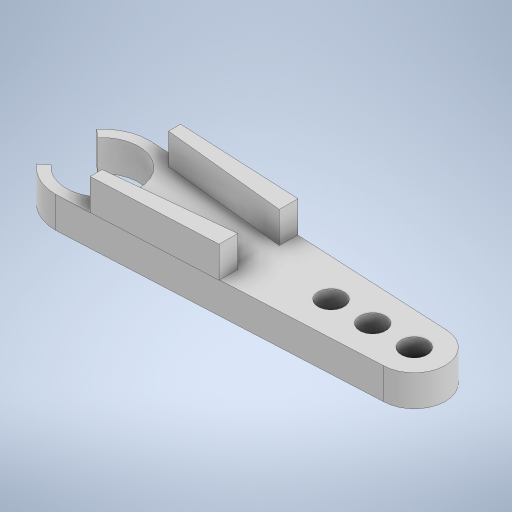
# Autodesk Inventor part: Servo Extension Clip-on
Saved by Autodesk Inventor 2023 (Build 270158000, 158)
## iProperties
Created: 2023-05-02
Part Number: Servo Extension Clip-on
Material: Generic
Document SubType Name: Modeling
Designer: adity
Density: 1 g/cm^3
Appearance: Default
Author: adity
Autodesk Inventor part; units mm, degrees
ref_plane "YZ Plane" through (0, 0, 0) normal (1, 0, 0) x (0, 1, 0)
ref_plane "XZ Plane" through (0, 0, 0) normal (0, 1, 0) x (-1, 0, 0)
ref_plane "XY Plane" through (0, 0, 0) normal (0, 0, 1) x (1, 0, 0)
sketch "Sketch2" plane through (0, 0, 0) normal (0, 1, 0) x (-1, 0, 0)
  circle A0 centre (0, 0) radius 3.5
  circle A1 centre (0, 0) radius 4.5
  line L0 (0, 0) -> (3.4472, 2.8925)
  line L1 (0, 0) -> (4.5, 0) construction
  line L2 (0, 0) -> (3.4472, -2.8925)
  line L3 (0, 0) -> (4.5, 0) construction
  line L4 (0, 0) -> (-30, 0)
  line L5 (0, 0) -> (30, 0) construction
  circle A2 centre (-30, 0) radius 1.25
  circle A3 centre (-26, 0) radius 1.25
  circle A4 centre (-22, 0) radius 1.25
  circle A5 centre (-30, 0) radius 3
  line L6 (0, 4.5) -> (-30, 3)
  line L7 (-0.0015, -4.5) -> (-30.1494, -2.9963)
  point P0 (2.6812, -2.2498)
  point P1 (2.6812, 2.2498)
  dimension "d11" = 7
  dimension "d12" = 9
  dimension "d13" = 40
  dimension "d14" = 40
  dimension "d15" = 30
  dimension "d16" = 180
  dimension "d17" = 2.5
  dimension "d20" = 4
  dimension "d25" = 6
  constraints: 16 end point, 6 centre point, 6 point on circle, 5 horizontal, 4 coincident, 3 equal length, 1 tangent, 4 other
  measures "d11" diameter of A0
  measures "d12" diameter of A1
  measures "d13" angle of L1 L0
  measures "d14" angle of L2 L3
  measures "d15" distance of L0.start L4.end
  measures "d16" angle of L4 L5
  measures "d17" diameter of A2
  measures "d20" distance of A2.centre A3.centre
  measures "d25" diameter of A5
extrude "Extrusion1" add sketch "Sketch2" along normal blind 3 contours A1 L4 A4 A3 A5 L6 | A0 L4 A1 L0 | L2 A1 L4 A0 | A1 L7 A5 A3 L4 A4 | A5 A3
sketch "Sketch4" plane through (0, 3, 0) normal (0, 1, 0) x (1, 0, 0)
  arc A0 (-2.6812, -2.2498) -> (-2.6812, 2.2498) centre (0, 0) ccw projected
  line L0 (0, 0) -> (15, 0)
  circle A1 centre (15, 0) radius 2
  circle A2 centre (0, 0) radius 3.5
  line L1 (15.0186, 1.9999) -> (0.3519, 3.4823)
  line L2 (15.0186, -1.9999) -> (0.3519, -3.4823)
  circle A3 centre (15, 0) radius 3.7945
  circle A4 centre (0, 0) radius 4.5
  line L3 (15.0186, 3.7945) -> (0.2127, 4.495)
  line L4 (15.0186, -3.7945) -> (0.2127, -4.495)
  line L5 (3.166, 3.1978) -> (3.166, 4.3552)
  line L6 (3.166, 3.1978) -> (4.3234, 3.1978) construction
  line L7 (3.166, -3.1978) -> (3.166, -4.3552)
  line L8 (3.166, -3.1978) -> (4.3234, -3.1978) construction
  line L9 (15.0186, 1.9999) -> (15.0186, 3.7945)
  line L10 (15.0186, -1.9999) -> (15.0186, -3.7945)
  dimension "d36" = 15
  dimension "d37" = 4
  dimension "d38" = 7
  dimension "d39" = 7.589
  dimension "d40" = 9
  dimension "d41" = 90
  dimension "d42" = 90
  constraints: 22 end point, 10 point on circle, 4 centre point, 4 coincident, 4 point on line, 4 tangent, 3 horizontal, 2 perpendicular, 2 vertical
  measures "d36" distance of L0.start L0.end
  measures "d37" diameter of A1
  measures "d38" diameter of A2
  measures "d39" diameter of A3
  measures "d40" diameter of A4
  measures "d41" angle of L6 L5
  measures "d42" angle of L7 L8
extrude "Extrusion2" add sketch "Sketch4" along normal blind 3 contours L2 A3 L4 L7 | L2 L10 A3 | L5 L3 A3 L1 | A3 L9 L1
body "Solid1"
